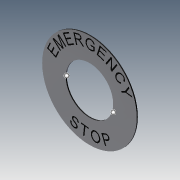
# Autodesk Inventor part: E-Stop Collar
Saved by Autodesk Inventor 2016 (Build 200138000, 138)
## iProperties
Created: 2005-06-20
Part Number: E-Stop Collar
Checked By: ~
Material: Generic
Document SubType Name: Modeling
Designer: BassBW
Manufacturer: Standard
Standards Organization: Custom
Density: 1 g/cm^3
Appearance: Black
SCALE: 1:1
STOCK SIZE: SEE DWG
UNITS: ANSI
COMMODITY: MFG
Author: BassBW
Autodesk Inventor part; units mm, degrees
ref_plane "YZ Plane" through (0, 0, 0) normal (1, 0, 0) x (0, 1, 0)
ref_plane "XZ Plane" through (0, 0, 0) normal (0, 1, 0) x (-1, 0, 0)
ref_plane "XY Plane" through (0, 0, 0) normal (0, 0, 1) x (1, 0, 0)
sketch "Sketch1" plane through (0, 0, 0) normal (0, 0, 1) x (1, 0, 0)
  circle A0 centre (0, 0) radius 29.972
  circle A1 centre (0, 0) radius 15
  dimension "d34" = 30
  dimension "d35" = 59.944
  constraints: 2 centre point, 2 coincident
  measures "d34" diameter of A1
  measures "d35" diameter of A0
extrude "Extrusion6" add sketch "Sketch1" along normal blind 0.635
sketch "Sketch10" plane through (0, 0, 0.635) normal (0, 0, 1) x (1, 0, 0)
  circle A0 centre (0, 0) radius 15 projected
  circle A1 centre (0, 0) radius 29.972 projected
  line L0 (0, 0) -> (0, 29.972) construction
  line L1 (0, 0) -> (-7.7573, 28.9507) construction
  line L2 (0, 0) -> (-14.986, 25.9565) construction
  line L3 (0, 0) -> (-21.1934, 21.1934) construction
  line L4 (0, 0) -> (-25.9565, 14.986) construction
  line L5 (0, 0) -> (-28.9507, 7.7573) construction
  line L6 (0, 0) -> (-29.972, 0) construction
  line L7 (0, 0) -> (-28.9507, -7.7573) construction
  line L8 (0, 0) -> (-25.9565, -14.986) construction
  line L9 (0, 0) -> (-21.1934, -21.1934) construction
  line L10 (0, 0) -> (-14.986, -25.9565) construction
  line L11 (0, 0) -> (-7.7573, -28.9507) construction
  line L12 (0, 0) -> (0, -29.972) construction
  line L13 (0, 0) -> (7.7573, -28.9507) construction
  line L14 (0, 0) -> (14.986, -25.9565) construction
  line L15 (0, 0) -> (21.1934, -21.1934) construction
  line L16 (0, 0) -> (25.9565, -14.986) construction
  line L17 (0, 0) -> (28.9507, -7.7573) construction
  line L18 (0, 0) -> (29.972, 0) construction
  line L19 (0, 0) -> (28.9507, 7.7573) construction
  line L20 (0, 0) -> (25.9565, 14.986) construction
  line L21 (0, 0) -> (21.1934, 21.1934) construction
  line L22 (0, 0) -> (14.986, 25.9565) construction
  line L23 (0, 0) -> (7.7573, 28.9507) construction
  circle A2 centre (0, 0) radius 20.6375 construction
  circle A3 centre (97.2399, -75.8106) radius 22.225 construction
  line L24 (-21.1834, 7.1074) -> (-26.9712, 9.7195)
  line L25 (-26.9712, 9.7195) -> (-25.1162, 13.8297)
  line L26 (-25.1162, 13.8297) -> (-24.4452, 13.5269)
  line L27 (-24.4452, 13.5269) -> (-25.9595, 10.1716)
  line L28 (-25.9595, 10.1716) -> (-24.1979, 9.3766)
  line L29 (-24.1979, 9.3766) -> (-22.7972, 12.4802)
  line L30 (-22.7972, 12.4802) -> (-22.1262, 12.1774)
  line L31 (-22.1262, 12.1774) -> (-23.5269, 9.0737)
  line L32 (-23.5269, 9.0737) -> (-21.5137, 8.1652)
  line L33 (-21.5137, 8.1652) -> (-19.9237, 11.6882)
  line L34 (-19.9237, 11.6882) -> (-19.2527, 11.3853)
  line L35 (-19.2527, 11.3853) -> (-21.1834, 7.1074)
  line L36 (-18.6254, 12.3234) -> (-23.3979, 16.5122)
  line L37 (-23.3979, 16.5122) -> (-22.5442, 17.4849)
  line L38 (-22.5442, 17.4849) -> (-18.2473, 15.5924)
  spline S0 degree 4 poles (-18.2473, 15.5924) (-18.2111, 15.5763) (-18.1401, 15.5449) (-18.0377, 15.4993) (-17.9095, 15.4421) (-17.7897, 15.3882) (-17.6783, 15.3378) (-17.5753, 15.2907) (-17.4806, 15.2471) (-17.4158, 15.217) (-17.3755, 15.198) (-17.356, 15.1888) knots 0 0 0 0 0 0.125 0.25 0.375 0.5 0.625 0.75 0.875 1 1 1 1 1
  spline S1 degree 4 poles (-17.356, 15.1888) (-17.3753, 15.1977) (-17.4137, 15.2188) (-17.4704, 15.2599) (-17.544, 15.3341) (-17.6157, 15.4274) (-17.6854, 15.5401) (-17.7533, 15.672) (-17.8191, 15.8231) (-17.8671, 15.9509) (-17.8984, 16.0425) (-17.9139, 16.0899) knots 0 0 0 0 0 0.125 0.25 0.375 0.5 0.625 0.75 0.875 1 1 1 1 1
  line L39 (-17.9139, 16.0899) -> (-20.3046, 20.0365)
  line L40 (-20.3046, 20.0365) -> (-19.4519, 21.008)
  line L41 (-19.4519, 21.008) -> (-14.6794, 16.8192)
  line L42 (-14.6794, 16.8192) -> (-15.2258, 16.1967)
  line L43 (-15.2258, 16.1967) -> (-19.3066, 19.7785)
  line L44 (-19.3066, 19.7785) -> (-16.3432, 14.9236)
  line L45 (-16.3432, 14.9236) -> (-16.9626, 14.2179)
  line L46 (-16.9626, 14.2179) -> (-22.1598, 16.5277)
  line L47 (-22.1598, 16.5277) -> (-18.079, 12.9459)
  line L48 (-18.079, 12.9459) -> (-18.6254, 12.3234)
  line L49 (-13.6101, 17.7205) -> (-16.9547, 23.1183)
  line L50 (-16.9547, 23.1183) -> (-13.1215, 25.4934)
  line L51 (-13.1215, 25.4934) -> (-12.7337, 24.8676)
  line L52 (-12.7337, 24.8676) -> (-15.8628, 22.9287)
  line L53 (-15.8628, 22.9287) -> (-14.8449, 21.2859)
  line L54 (-14.8449, 21.2859) -> (-11.9505, 23.0793)
  line L55 (-11.9505, 23.0793) -> (-11.5627, 22.4535)
  line L56 (-11.5627, 22.4535) -> (-14.4572, 20.66)
  line L57 (-14.4572, 20.66) -> (-13.2938, 18.7825)
  line L58 (-13.2938, 18.7825) -> (-10.0082, 20.8184)
  line L59 (-10.0082, 20.8184) -> (-9.6204, 20.1925)
  line L60 (-9.6204, 20.1925) -> (-13.6101, 17.7205)
  line L61 (-8.4915, 20.6592) -> (-10.2418, 26.7632)
  line L62 (-10.2418, 26.7632) -> (-7.6307, 27.5119)
  spline S2 degree 4 poles (-7.6307, 27.5119) (-7.5837, 27.5279) (-7.4887, 27.5575) (-7.3437, 27.5947) (-7.1453, 27.6296) (-6.9424, 27.6495) (-6.7362, 27.6533) (-6.529, 27.639) (-6.3241, 27.604) (-6.1251, 27.5462) (-5.936, 27.4647) (-5.7602, 27.361) (-5.6004, 27.2395) (-5.4589, 27.1057) (-5.3372, 26.9653) (-5.2365, 26.8227) (-5.1572, 26.6804) (-5.114, 26.5746) (-5.0925, 26.5046) (-5.0835, 26.4697) knots 0 0 0 0 0 0.0625 0.125 0.1875 0.25 0.3125 0.375 0.4375 0.5 0.5625 0.625 0.6875 0.75 0.8125 0.875 0.9375 1 1 1 1 1
  spline S3 degree 4 poles (-5.0835, 26.4697) (-5.0692, 26.4244) (-5.0454, 26.3325) (-5.0248, 26.1909) (-5.0273, 25.9947) (-5.0593, 25.7922) (-5.1197, 25.5855) (-5.2066, 25.3784) (-5.3175, 25.1763) (-5.4496, 24.9849) (-5.6002, 24.8093) (-5.7677, 24.6532) (-5.951, 24.5185) (-6.1001, 24.4343) (-6.2046, 24.3857) (-6.2581, 24.3632) knots 0 0 0 0 0 0.083333 0.166667 0.25 0.333333 0.416667 0.5 0.583333 0.666667 0.75 0.833333 0.916667 1 1 1 1 1
  spline S4 degree 4 poles (-6.2581, 24.3632) (-6.2373, 24.3584) (-6.1963, 24.3485) (-6.1368, 24.333) (-6.0616, 24.3112) (-5.9906, 24.2882) (-5.9236, 24.264) (-5.8608, 24.2386) (-5.802, 24.2121) (-5.7611, 24.1913) (-5.7351, 24.177) (-5.7225, 24.1698) knots 0 0 0 0 0 0.125 0.25 0.375 0.5 0.625 0.75 0.875 1 1 1 1 1
  spline S5 degree 4 poles (-5.7225, 24.1698) (-5.696, 24.1538) (-5.6431, 24.1213) (-5.5636, 24.0704) (-5.4573, 23.9985) (-5.3509, 23.9226) (-5.2442, 23.8427) (-5.1373, 23.7588) (-5.0302, 23.6708) (-4.9496, 23.6018) (-4.8959, 23.5544) (-4.869, 23.5304) knots 0 0 0 0 0 0.125 0.25 0.375 0.5 0.625 0.75 0.875 1 1 1 1 1
  line L63 (-4.869, 23.5304) -> (-3.3841, 22.1238)
  line L64 (-3.3841, 22.1238) -> (-4.2964, 21.8622)
  line L65 (-4.2964, 21.8622) -> (-5.4387, 22.9348)
  spline S6 degree 4 poles (-5.4387, 22.9348) (-5.4676, 22.9622) (-5.526, 23.017) (-5.6152, 23.0989) (-5.7369, 23.2072) (-5.8614, 23.3143) (-5.9881, 23.4194) (-6.1159, 23.5208) (-6.2435, 23.6163) (-6.369, 23.7031) (-6.4906, 23.7791) (-6.6065, 23.8426) (-6.7153, 23.8935) (-6.8159, 23.9324) (-6.9074, 23.9604) (-6.9893, 23.9785) (-7.0613, 23.9875) (-7.1077, 23.9875) (-7.1353, 23.9846) (-7.1482, 23.9823) knots 0 0 0 0 0 0.0625 0.125 0.1875 0.25 0.3125 0.375 0.4375 0.5 0.5625 0.625 0.6875 0.75 0.8125 0.875 0.9375 1 1 1 1 1
  spline S7 degree 4 poles (-7.1482, 23.9823) (-7.1586, 23.9798) (-7.1799, 23.9747) (-7.2135, 23.9667) (-7.2616, 23.9557) (-7.313, 23.9442) (-7.3677, 23.9322) (-7.4258, 23.9198) (-7.4871, 23.907) (-7.5356, 23.897) (-7.569, 23.8902) (-7.586, 23.8867) knots 0 0 0 0 0 0.125 0.25 0.375 0.5 0.625 0.75 0.875 1 1 1 1 1
  line L66 (-7.586, 23.8867) -> (-8.4817, 23.6299)
  line L67 (-8.4817, 23.6299) -> (-7.6953, 20.8875)
  line L68 (-7.6953, 20.8875) -> (-8.4915, 20.6592)
  line L69 (-8.6846, 24.3376) -> (-7.0245, 24.8136)
  spline S8 degree 4 poles (-7.0245, 24.8136) (-6.9917, 24.8213) (-6.9261, 24.8385) (-6.8282, 24.8693) (-6.6986, 24.9205) (-6.5704, 24.9818) (-6.445, 25.0533) (-6.3244, 25.1348) (-6.2119, 25.2263) (-6.1109, 25.3273) (-6.0242, 25.4364) (-5.9537, 25.5514) (-5.8999, 25.669) (-5.8623, 25.7854) (-5.8397, 25.8968) (-5.8313, 26.0006) (-5.8366, 26.0952) (-5.8507, 26.1588) (-5.8645, 26.1978) (-5.8726, 26.2165) knots 0 0 0 0 0 0.0625 0.125 0.1875 0.25 0.3125 0.375 0.4375 0.5 0.5625 0.625 0.6875 0.75 0.8125 0.875 0.9375 1 1 1 1 1
  spline S9 degree 4 poles (-5.8726, 26.2165) (-5.8806, 26.2463) (-5.9003, 26.3044) (-5.9407, 26.3873) (-6.0164, 26.4895) (-6.113, 26.5828) (-6.2292, 26.6666) (-6.3621, 26.7393) (-6.5079, 26.7989) (-6.6626, 26.8433) (-6.8226, 26.8706) (-6.9851, 26.8795) (-7.149, 26.8693) (-7.2724, 26.847) (-7.3548, 26.8256) (-7.396, 26.8133) knots 0 0 0 0 0 0.083333 0.166667 0.25 0.333333 0.416667 0.5 0.583333 0.666667 0.75 0.833333 0.916667 1 1 1 1 1
  line L70 (-7.396, 26.8133) -> (-9.2427, 26.2838)
  line L71 (-9.2427, 26.2838) -> (-8.6846, 24.3376)
  line L72 (0.6669, 24.634) -> (0.6809, 25.3701)
  line L73 (0.6809, 25.3701) -> (3.3493, 25.3194)
  line L74 (3.3493, 25.3194) -> (3.305, 22.9889)
  spline S10 degree 4 poles (3.305, 22.9889) (3.2625, 22.9569) (3.1749, 22.8937) (3.0352, 22.8014) (2.8324, 22.6835) (2.6141, 22.571) (2.3821, 22.4647) (2.1402, 22.3663) (1.8933, 22.2778) (1.6469, 22.2015) (1.4061, 22.1397) (1.1745, 22.0938) (0.9543, 22.0647) (0.7983, 22.0559) (0.6985, 22.0557) (0.6496, 22.0571) knots 0 0 0 0 0 0.083333 0.166667 0.25 0.333333 0.416667 0.5 0.583333 0.666667 0.75 0.833333 0.916667 1 1 1 1 1
  spline S11 degree 4 poles (0.6496, 22.0571) (0.5839, 22.0551) (0.4507, 22.0568) (0.2456, 22.0764) (-0.0381, 22.1364) (-0.3308, 22.2304) (-0.6292, 22.3583) (-0.9272, 22.5201) (-1.2169, 22.7155) (-1.4897, 22.9429) (-1.7378, 23.1991) (-1.9557, 23.4786) (-2.1405, 23.7734) (-2.291, 24.0752) (-2.4074, 24.3759) (-2.4897, 24.6698) (-2.5383, 24.9536) (-2.5495, 25.1579) (-2.5457, 25.2901) (-2.5409, 25.3552) knots 0 0 0 0 0 0.0625 0.125 0.1875 0.25 0.3125 0.375 0.4375 0.5 0.5625 0.625 0.6875 0.75 0.8125 0.875 0.9375 1 1 1 1 1
  spline S12 degree 4 poles (-2.5409, 25.3552) (-2.5425, 25.4202) (-2.5402, 25.5524) (-2.5206, 25.7569) (-2.4621, 26.042) (-2.3712, 26.3378) (-2.2477, 26.6409) (-2.0915, 26.945) (-1.9025, 27.2414) (-1.6819, 27.521) (-1.4324, 27.7755) (-1.1592, 27.9988) (-0.8697, 28.188) (-0.5722, 28.3417) (-0.2742, 28.4601) (0.0186, 28.5433) (0.303, 28.5915) (0.509, 28.6015) (0.643, 28.5966) (0.7091, 28.5912) knots 0 0 0 0 0 0.0625 0.125 0.1875 0.25 0.3125 0.375 0.4375 0.5 0.5625 0.625 0.6875 0.75 0.8125 0.875 0.9375 1 1 1 1 1
  spline S13 degree 4 poles (0.7091, 28.5912) (0.7554, 28.5917) (0.8495, 28.5899) (0.9953, 28.5783) (1.1987, 28.5451) (1.4103, 28.4942) (1.6279, 28.4251) (1.8477, 28.3376) (2.0645, 28.2311) (2.2726, 28.1058) (2.4667, 27.9625) (2.643, 27.8038) (2.7992, 27.6333) (2.9346, 27.4554) (3.0488, 27.2741) (3.1419, 27.0926) (3.214, 26.9124) (3.2522, 26.7789) (3.2707, 26.6907) (3.2782, 26.6468) knots 0 0 0 0 0 0.0625 0.125 0.1875 0.25 0.3125 0.375 0.4375 0.5 0.5625 0.625 0.6875 0.75 0.8125 0.875 0.9375 1 1 1 1 1
  line L75 (3.2782, 26.6468) -> (2.5123, 26.4542)
  spline S14 degree 4 poles (2.5123, 26.4542) (2.5056, 26.4862) (2.4899, 26.5504) (2.4597, 26.6473) (2.4058, 26.7773) (2.3383, 26.9079) (2.257, 27.0378) (2.1614, 27.165) (2.0514, 27.2868) (1.927, 27.4004) (1.7896, 27.5031) (1.6418, 27.5933) (1.4874, 27.6702) (1.3307, 27.7337) (1.1757, 27.7839) (1.0255, 27.8212) (0.8817, 27.8455) (0.7791, 27.8542) (0.7131, 27.8557) (0.6807, 27.8554) knots 0 0 0 0 0 0.0625 0.125 0.1875 0.25 0.3125 0.375 0.4375 0.5 0.5625 0.625 0.6875 0.75 0.8125 0.875 0.9375 1 1 1 1 1
  spline S15 degree 4 poles (0.6807, 27.8554) (0.6432, 27.8573) (0.5672, 27.859) (0.45, 27.8549) (0.2875, 27.8363) (0.1195, 27.8045) (-0.0528, 27.7596) (-0.2269, 27.7014) (-0.3994, 27.6299) (-0.5666, 27.5458) (-0.7247, 27.4499) (-0.8707, 27.3446) (-1.0028, 27.2328) (-1.1196, 27.1182) (-1.2206, 27.004) (-1.3054, 26.893) (-1.3738, 26.7864) (-1.4128, 26.7103) (-1.4333, 26.6614) (-1.4422, 26.6373) knots 0 0 0 0 0 0.0625 0.125 0.1875 0.25 0.3125 0.375 0.4375 0.5 0.5625 0.625 0.6875 0.75 0.8125 0.875 0.9375 1 1 1 1 1
  spline S16 degree 4 poles (-1.4422, 26.6373) (-1.4583, 26.6008) (-1.4893, 26.5272) (-1.5319, 26.4153) (-1.581, 26.2631) (-1.6224, 26.1079) (-1.6561, 25.9496) (-1.6822, 25.7883) (-1.7006, 25.6239) (-1.7087, 25.4984) (-1.7115, 25.4137) (-1.7122, 25.3711) knots 0 0 0 0 0 0.125 0.25 0.375 0.5 0.625 0.75 0.875 1 1 1 1 1
  spline S17 degree 4 poles (-1.7122, 25.3711) (-1.7163, 25.3156) (-1.7204, 25.2038) (-1.7142, 25.0334) (-1.6811, 24.8007) (-1.6231, 24.5636) (-1.5401, 24.3244) (-1.4316, 24.0873) (-1.2972, 23.8581) (-1.1377, 23.6431) (-0.9548, 23.4479) (-0.7528, 23.2766) (-0.5382, 23.1311) (-0.318, 23.0118) (-0.0992, 22.9183) (0.1131, 22.8502) (0.3158, 22.8071) (0.4598, 22.7935) (0.5522, 22.7927) (0.5974, 22.7944) knots 0 0 0 0 0 0.0625 0.125 0.1875 0.25 0.3125 0.375 0.4375 0.5 0.5625 0.625 0.6875 0.75 0.8125 0.875 0.9375 1 1 1 1 1
  spline S18 degree 4 poles (0.5974, 22.7944) (0.6354, 22.7941) (0.7128, 22.7956) (0.8335, 22.8043) (1.0033, 22.8289) (1.1812, 22.866) (1.3651, 22.9145) (1.5514, 22.9727) (1.7349, 23.038) (1.9102, 23.1074) (2.0719, 23.1784) (2.2161, 23.249) (2.3407, 23.318) (2.4188, 23.3682) (2.4639, 23.401) (2.4847, 23.4172) knots 0 0 0 0 0 0.083333 0.166667 0.25 0.333333 0.416667 0.5 0.583333 0.666667 0.75 0.833333 0.916667 1 1 1 1 1
  line L76 (2.4847, 23.4172) -> (2.5072, 24.599)
  line L77 (2.5072, 24.599) -> (0.6669, 24.634)
  line L78 (4.5777, 21.87) -> (6.494, 27.9239)
  line L79 (6.494, 27.9239) -> (10.7932, 26.563)
  line L80 (10.7932, 26.563) -> (10.571, 25.8611)
  line L81 (10.571, 25.8611) -> (7.0614, 26.972)
  line L82 (7.0614, 26.972) -> (6.4782, 25.1295)
  line L83 (6.4782, 25.1295) -> (9.7245, 24.1019)
  line L84 (9.7245, 24.1019) -> (9.5023, 23.4)
  line L85 (9.5023, 23.4) -> (6.256, 24.4276)
  line L86 (6.256, 24.4276) -> (5.5895, 22.3219)
  line L87 (5.5895, 22.3219) -> (9.2745, 21.1554)
  line L88 (9.2745, 21.1554) -> (9.0523, 20.4535)
  line L89 (9.0523, 20.4535) -> (4.5777, 21.87)
  line L90 (10.1418, 19.901) -> (13.6325, 25.2055)
  line L91 (13.6325, 25.2055) -> (14.3689, 24.721)
  line L92 (14.3689, 24.721) -> (14.3133, 18.8739)
  line L93 (14.3133, 18.8739) -> (17.0151, 22.9796)
  line L94 (17.0151, 22.9796) -> (17.707, 22.5243)
  line L95 (17.707, 22.5243) -> (14.2163, 17.2198)
  line L96 (14.2163, 17.2198) -> (13.4799, 17.7043)
  line L97 (13.4799, 17.7043) -> (13.5355, 23.5514)
  line L98 (13.5355, 23.5514) -> (10.8337, 19.4457)
  line L99 (10.8337, 19.4457) -> (10.1418, 19.901)
  line L100 (19.8442, 14.3837) -> (20.2195, 13.6161)
  spline S19 degree 4 poles (20.2195, 13.6161) (20.1553, 13.5829) (20.0244, 13.5217) (19.8209, 13.4461) (19.5351, 13.3772) (19.2365, 13.3403) (18.9278, 13.3346) (18.6145, 13.3595) (18.3041, 13.4135) (18.0049, 13.4952) (17.7245, 13.6034) (17.4684, 13.7371) (17.2398, 13.8958) (17.0899, 14.0334) (16.9996, 14.1333) (16.9569, 14.1854) knots 0 0 0 0 0 0.083333 0.166667 0.25 0.333333 0.416667 0.5 0.583333 0.666667 0.75 0.833333 0.916667 1 1 1 1 1
  spline S20 degree 4 poles (16.9569, 14.1854) (16.9098, 14.2339) (16.8201, 14.3354) (16.699, 14.5007) (16.5646, 14.747) (16.4579, 15.0182) (16.3804, 15.3122) (16.3346, 15.6249) (16.324, 15.9508) (16.3508, 16.2833) (16.4157, 16.6155) (16.516, 16.9404) (16.6459, 17.2517) (16.7984, 17.5441) (16.9662, 17.8129) (17.1442, 18.0553) (17.3294, 18.2693) (17.4728, 18.4082) (17.5702, 18.491) (17.6194, 18.53) knots 0 0 0 0 0 0.0625 0.125 0.1875 0.25 0.3125 0.375 0.4375 0.5 0.5625 0.625 0.6875 0.75 0.8125 0.875 0.9375 1 1 1 1 1
  spline S21 degree 4 poles (17.6194, 18.53) (17.668, 18.575) (17.7694, 18.6624) (17.9344, 18.7851) (18.18, 18.9321) (18.4503, 19.0616) (18.7432, 19.1716) (19.0551, 19.2586) (19.3807, 19.3178) (19.7136, 19.3448) (20.0468, 19.3368) (20.373, 19.2937) (20.6851, 19.2186) (20.9768, 19.1166) (21.2427, 18.993) (21.4789, 18.852) (21.6834, 18.696) (21.8123, 18.5685) (21.8872, 18.4789) (21.922, 18.433) knots 0 0 0 0 0 0.0625 0.125 0.1875 0.25 0.3125 0.375 0.4375 0.5 0.5625 0.625 0.6875 0.75 0.8125 0.875 0.9375 1 1 1 1 1
  spline S22 degree 4 poles (21.922, 18.433) (21.9634, 18.3857) (22.042, 18.2874) (22.1471, 18.1291) (22.2616, 17.8966) (22.3506, 17.6439) (22.414, 17.3738) (22.4517, 17.0914) (22.4634, 16.8038) (22.4491, 16.5186) (22.4086, 16.243) (22.3419, 15.9821) (22.2488, 15.7386) (22.1592, 15.57) (22.0907, 15.4639) (22.0542, 15.4124) knots 0 0 0 0 0 0.083333 0.166667 0.25 0.333333 0.416667 0.5 0.583333 0.666667 0.75 0.833333 0.916667 1 1 1 1 1
  line L101 (22.0542, 15.4124) -> (21.3717, 15.9197)
  spline S23 degree 4 poles (21.3717, 15.9197) (21.3985, 15.9587) (21.449, 16.0383) (21.5155, 16.1625) (21.5856, 16.3374) (21.6373, 16.5208) (21.6705, 16.7111) (21.6853, 16.9052) (21.6819, 17.099) (21.6603, 17.2878) (21.6205, 17.4674) (21.5628, 17.6344) (21.4871, 17.7873) (21.4169, 17.8908) (21.364, 17.9548) (21.3361, 17.9855) knots 0 0 0 0 0 0.083333 0.166667 0.25 0.333333 0.416667 0.5 0.583333 0.666667 0.75 0.833333 0.916667 1 1 1 1 1
  spline S24 degree 4 poles (21.3361, 17.9855) (21.3077, 18.0237) (21.2469, 18.0971) (21.1436, 18.1987) (20.9819, 18.3167) (20.797, 18.4167) (20.5906, 18.4976) (20.3662, 18.5568) (20.1282, 18.5917) (19.882, 18.5996) (19.6336, 18.5798) (19.3884, 18.5338) (19.1516, 18.4659) (18.9279, 18.3812) (18.7207, 18.285) (18.5327, 18.1815) (18.3653, 18.0727) (18.2555, 17.988) (18.1895, 17.9302) (18.1582, 17.9009) knots 0 0 0 0 0 0.0625 0.125 0.1875 0.25 0.3125 0.375 0.4375 0.5 0.5625 0.625 0.6875 0.75 0.8125 0.875 0.9375 1 1 1 1 1
  spline S25 degree 4 poles (18.1582, 17.9009) (18.117, 17.8691) (18.0354, 17.8021) (17.9161, 17.6918) (17.763, 17.5253) (17.6169, 17.3397) (17.4799, 17.1361) (17.3557, 16.9166) (17.2496, 16.6839) (17.1667, 16.4419) (17.1112, 16.1951) (17.0849, 15.9491) (17.0865, 15.7095) (17.1131, 15.4823) (17.161, 15.2725) (17.2272, 15.084) (17.31, 14.9188) (17.3841, 14.8131) (17.4387, 14.7508) (17.4674, 14.7217) knots 0 0 0 0 0 0.0625 0.125 0.1875 0.25 0.3125 0.375 0.4375 0.5 0.5625 0.625 0.6875 0.75 0.8125 0.875 0.9375 1 1 1 1 1
  spline S26 degree 4 poles (17.4674, 14.7217) (17.4974, 14.6848) (17.5611, 14.614) (17.6679, 14.517) (17.8321, 14.406) (18.0173, 14.3136) (18.2212, 14.2401) (18.4395, 14.1863) (18.6665, 14.1531) (18.896, 14.1417) (19.1223, 14.1529) (19.3415, 14.1876) (19.5512, 14.2461) (19.7008, 14.3079) (19.797, 14.3571) (19.8442, 14.3837) knots 0 0 0 0 0 0.083333 0.166667 0.25 0.333333 0.416667 0.5 0.583333 0.666667 0.75 0.833333 0.916667 1 1 1 1 1
  line L102 (20.0309, 9.6686) -> (22.4765, 10.7899)
  line L103 (22.4765, 10.7899) -> (24.8059, 14.4901)
  line L104 (24.8059, 14.4901) -> (25.2104, 13.6078)
  line L105 (25.2104, 13.6078) -> (23.99, 11.6705)
  spline S27 degree 4 poles (23.99, 11.6705) (23.9679, 11.6348) (23.9242, 11.5644) (23.86, 11.461) (23.777, 11.3281) (23.6966, 11.1999) (23.6189, 11.0765) (23.5439, 10.9578) (23.4716, 10.844) (23.4193, 10.7622) (23.3853, 10.7093) (23.3686, 10.6832) knots 0 0 0 0 0 0.125 0.25 0.375 0.5 0.625 0.75 0.875 1 1 1 1 1
  spline S28 degree 4 poles (23.3686, 10.6832) (23.3977, 10.6782) (23.4572, 10.6682) (23.5508, 10.6534) (23.684, 10.6341) (23.8256, 10.6153) (23.9756, 10.5968) (24.1341, 10.5789) (24.3009, 10.5613) (24.4324, 10.5485) (24.5228, 10.54) (24.5688, 10.5359) knots 0 0 0 0 0 0.125 0.25 0.375 0.5 0.625 0.75 0.875 1 1 1 1 1
  line L106 (24.5688, 10.5359) -> (26.741, 10.2695)
  line L107 (26.741, 10.2695) -> (27.1455, 9.3871)
  line L108 (27.1455, 9.3871) -> (22.8217, 10.037)
  line L109 (22.8217, 10.037) -> (20.3761, 8.9157)
  line L110 (20.3761, 8.9157) -> (20.0309, 9.6686)
  circle A4 centre (97.2399, -80.7117) radius 22.225 construction
  line L111 (-12.1327, -22.3139) -> (-11.351, -22.5876)
  spline S29 degree 4 poles (-11.351, -22.5876) (-11.3611, -22.6199) (-11.379, -22.6859) (-11.3987, -22.7891) (-11.4105, -22.935) (-11.4076, -23.0886) (-11.3893, -23.2488) (-11.3544, -23.4132) (-11.3012, -23.5788) (-11.2288, -23.742) (-11.1374, -23.8992) (-11.0289, -24.0474) (-10.9072, -24.1839) (-10.7766, -24.3069) (-10.6417, -24.4147) (-10.5054, -24.5064) (-10.3697, -24.5816) (-10.2688, -24.6253) (-10.2021, -24.6488) (-10.1688, -24.6591) knots 0 0 0 0 0 0.0625 0.125 0.1875 0.25 0.3125 0.375 0.4375 0.5 0.5625 0.625 0.6875 0.75 0.8125 0.875 0.9375 1 1 1 1 1
  spline S30 degree 4 poles (-10.1688, -24.6591) (-10.1411, -24.6702) (-10.0842, -24.6908) (-9.9943, -24.7169) (-9.8652, -24.7423) (-9.7277, -24.7579) (-9.5829, -24.7633) (-9.4333, -24.7575) (-9.2823, -24.7393) (-9.1336, -24.7075) (-8.9912, -24.662) (-8.8587, -24.6038) (-8.7387, -24.5355) (-8.6333, -24.4602) (-8.5439, -24.3813) (-8.4716, -24.3014) (-8.4168, -24.2218) (-8.3891, -24.1628) (-8.3766, -24.1239) (-8.3718, -24.1045) knots 0 0 0 0 0 0.0625 0.125 0.1875 0.25 0.3125 0.375 0.4375 0.5 0.5625 0.625 0.6875 0.75 0.8125 0.875 0.9375 1 1 1 1 1
  spline S31 degree 4 poles (-8.3718, -24.1045) (-8.3646, -24.0864) (-8.3521, -24.0491) (-8.3391, -23.9903) (-8.3333, -23.906) (-8.3389, -23.8163) (-8.3555, -23.722) (-8.3826, -23.6247) (-8.4194, -23.5268) (-8.4649, -23.4304) (-8.5185, -23.3379) (-8.5794, -23.2508) (-8.6475, -23.1699) (-8.7038, -23.1141) (-8.7436, -23.0791) (-8.7641, -23.0622) knots 0 0 0 0 0 0.083333 0.166667 0.25 0.333333 0.416667 0.5 0.583333 0.666667 0.75 0.833333 0.916667 1 1 1 1 1
  spline S32 degree 4 poles (-8.7641, -23.0622) (-8.7846, -23.0459) (-8.8302, -23.0107) (-8.9122, -22.9494) (-9.0483, -22.8509) (-9.2096, -22.7368) (-9.3924, -22.6089) (-9.5899, -22.4711) (-9.7932, -22.3284) (-9.9926, -22.1862) (-10.1792, -22.0493) (-10.3466, -21.9215) (-10.4911, -21.8048) (-10.5813, -21.7261) (-10.6332, -21.6776) (-10.6571, -21.6544) knots 0 0 0 0 0 0.083333 0.166667 0.25 0.333333 0.416667 0.5 0.583333 0.666667 0.75 0.833333 0.916667 1 1 1 1 1
  spline S33 degree 4 poles (-10.6571, -21.6544) (-10.681, -21.6298) (-10.7275, -21.5786) (-10.7925, -21.4962) (-10.8699, -21.375) (-10.9379, -21.2431) (-10.9961, -21.1018) (-11.044, -20.9538) (-11.0808, -20.8026) (-11.1056, -20.652) (-11.1177, -20.5057) (-11.1164, -20.3663) (-11.1014, -20.2352) (-11.0798, -20.1435) (-11.0607, -20.0855) (-11.0501, -20.0572) knots 0 0 0 0 0 0.083333 0.166667 0.25 0.333333 0.416667 0.5 0.583333 0.666667 0.75 0.833333 0.916667 1 1 1 1 1
  spline S34 degree 4 poles (-11.0501, -20.0572) (-11.041, -20.0238) (-11.0187, -19.9572) (-10.9725, -19.8576) (-10.8853, -19.7256) (-10.7731, -19.5953) (-10.6368, -19.4687) (-10.4779, -19.3494) (-10.299, -19.2419) (-10.1032, -19.1507) (-9.8947, -19.0793) (-9.6785, -19.029) (-9.4602, -18.9993) (-9.2451, -18.9883) (-9.0379, -18.994) (-8.8421, -19.0147) (-8.6593, -19.0496) (-8.5327, -19.086) (-8.453, -19.1149) (-8.4144, -19.1305) knots 0 0 0 0 0 0.0625 0.125 0.1875 0.25 0.3125 0.375 0.4375 0.5 0.5625 0.625 0.6875 0.75 0.8125 0.875 0.9375 1 1 1 1 1
  spline S35 degree 4 poles (-8.4144, -19.1305) (-8.3705, -19.1435) (-8.2827, -19.1731) (-8.1504, -19.2279) (-7.973, -19.3214) (-7.7956, -19.4354) (-7.6201, -19.5694) (-7.4504, -19.7227) (-7.2915, -19.8939) (-7.1488, -20.0812) (-7.027, -20.2814) (-6.929, -20.4905) (-6.8555, -20.703) (-6.806, -20.9132) (-6.7792, -21.1161) (-6.7739, -21.3078) (-6.7895, -21.4861) (-6.8166, -21.6092) (-6.8416, -21.6864) (-6.8557, -21.7238) knots 0 0 0 0 0 0.0625 0.125 0.1875 0.25 0.3125 0.375 0.4375 0.5 0.5625 0.625 0.6875 0.75 0.8125 0.875 0.9375 1 1 1 1 1
  line L112 (-6.8557, -21.7238) -> (-7.6375, -21.4501)
  spline S36 degree 4 poles (-7.6375, -21.4501) (-7.6264, -21.4105) (-7.6083, -21.3309) (-7.5935, -21.2106) (-7.5983, -21.0485) (-7.6273, -20.8854) (-7.6797, -20.7226) (-7.7537, -20.5628) (-7.8473, -20.4098) (-7.958, -20.2675) (-8.0838, -20.1395) (-8.2229, -20.0284) (-8.3747, -19.9355) (-8.4977, -19.8801) (-8.5838, -19.8495) (-8.6278, -19.8358) knots 0 0 0 0 0 0.083333 0.166667 0.25 0.333333 0.416667 0.5 0.583333 0.666667 0.75 0.833333 0.916667 1 1 1 1 1
  spline S37 degree 4 poles (-8.6278, -19.8358) (-8.6709, -19.8196) (-8.7573, -19.7904) (-8.8869, -19.7565) (-9.0597, -19.7307) (-9.2318, -19.7242) (-9.4018, -19.7363) (-9.5667, -19.7658) (-9.7227, -19.811) (-9.8653, -19.8702) (-9.9901, -19.9416) (-10.0941, -20.0238) (-10.1755, -20.1162) (-10.219, -20.1929) (-10.2402, -20.2473) (-10.2488, -20.2753) knots 0 0 0 0 0 0.083333 0.166667 0.25 0.333333 0.416667 0.5 0.583333 0.666667 0.75 0.833333 0.916667 1 1 1 1 1
  spline S38 degree 4 poles (-10.2488, -20.2753) (-10.2559, -20.2954) (-10.2687, -20.3355) (-10.2838, -20.395) (-10.2957, -20.4733) (-10.2995, -20.5504) (-10.295, -20.6264) (-10.2824, -20.7013) (-10.2616, -20.7751) (-10.2399, -20.8296) (-10.2227, -20.8655) (-10.2134, -20.8834) knots 0 0 0 0 0 0.125 0.25 0.375 0.5 0.625 0.75 0.875 1 1 1 1 1
  spline S39 degree 4 poles (-10.2134, -20.8834) (-10.1946, -20.9084) (-10.1511, -20.9609) (-10.0687, -21.047) (-9.9246, -21.1762) (-9.7483, -21.3189) (-9.5443, -21.473) (-9.3206, -21.6346) (-9.0883, -21.7985) (-8.8589, -21.9591) (-8.6432, -22.1114) (-8.449, -22.2515) (-8.2806, -22.3774) (-8.175, -22.4606) (-8.114, -22.5109) (-8.0858, -22.5348) knots 0 0 0 0 0 0.083333 0.166667 0.25 0.333333 0.416667 0.5 0.583333 0.666667 0.75 0.833333 0.916667 1 1 1 1 1
  spline S40 degree 4 poles (-8.0858, -22.5348) (-8.0561, -22.5623) (-7.9985, -22.6193) (-7.9177, -22.7114) (-7.8212, -22.8471) (-7.7359, -22.9951) (-7.6624, -23.1537) (-7.6013, -23.3203) (-7.5538, -23.491) (-7.5208, -23.6614) (-7.5036, -23.8278) (-7.5027, -23.987) (-7.5187, -24.1377) (-7.5435, -24.2437) (-7.5657, -24.3113) (-7.5782, -24.3443) knots 0 0 0 0 0 0.083333 0.166667 0.25 0.333333 0.416667 0.5 0.583333 0.666667 0.75 0.833333 0.916667 1 1 1 1 1
  spline S41 degree 4 poles (-7.5782, -24.3443) (-7.588, -24.3793) (-7.612, -24.4494) (-7.6616, -24.5544) (-7.7547, -24.694) (-7.8745, -24.8323) (-8.0198, -24.9673) (-8.1889, -25.0954) (-8.3791, -25.2118) (-8.5869, -25.3119) (-8.8081, -25.3919) (-9.0372, -25.4503) (-9.2686, -25.4873) (-9.4966, -25.5042) (-9.7163, -25.5027) (-9.9245, -25.4843) (-10.119, -25.4497) (-10.2542, -25.4119) (-10.3395, -25.3815) (-10.3809, -25.3649) knots 0 0 0 0 0 0.0625 0.125 0.1875 0.25 0.3125 0.375 0.4375 0.5 0.5625 0.625 0.6875 0.75 0.8125 0.875 0.9375 1 1 1 1 1
  spline S42 degree 4 poles (-10.3809, -25.3649) (-10.4341, -25.3493) (-10.5404, -25.3141) (-10.6988, -25.2496) (-10.9081, -25.1399) (-11.1146, -25.0069) (-11.3159, -24.8509) (-11.5083, -24.6726) (-11.6862, -24.4732) (-11.8442, -24.2547) (-11.9772, -24.0204) (-12.0826, -23.7752) (-12.1599, -23.5252) (-12.2101, -23.2773) (-12.2349, -23.0374) (-12.2357, -22.8101) (-12.2135, -22.598) (-12.1797, -22.4511) (-12.1496, -22.3587) (-12.1327, -22.3139) knots 0 0 0 0 0 0.0625 0.125 0.1875 0.25 0.3125 0.375 0.4375 0.5 0.5625 0.625 0.6875 0.75 0.8125 0.875 0.9375 1 1 1 1 1
  line L113 (-4.0735, -26.7652) -> (-3.4252, -21.189)
  line L114 (-3.4252, -21.189) -> (-5.5277, -20.9446)
  line L115 (-5.5277, -20.9446) -> (-5.4426, -20.2133)
  line L116 (-5.4426, -20.2133) -> (-0.4149, -20.7978)
  line L117 (-0.4149, -20.7978) -> (-0.4999, -21.5291)
  line L118 (-0.4999, -21.5291) -> (-2.6024, -21.2847)
  line L119 (-2.6024, -21.2847) -> (-3.2508, -26.8609)
  line L120 (-3.2508, -26.8609) -> (-4.0735, -26.7652)
  spline S43 degree 4 poles (0.872, -23.9984) (0.8563, -23.8936) (0.8342, -23.6845) (0.8293, -23.372) (0.8788, -22.9581) (0.9832, -22.5485) (1.14, -22.1473) (1.3442, -21.7614) (1.5893, -21.4007) (1.8677, -21.0762) (2.1726, -20.7979) (2.499, -20.5734) (2.844, -20.4067) (3.1158, -20.3264) (3.3028, -20.2929) (3.3977, -20.2811) knots 0 0 0 0 0 0.083333 0.166667 0.25 0.333333 0.416667 0.5 0.583333 0.666667 0.75 0.833333 0.916667 1 1 1 1 1
  spline S44 degree 4 poles (3.3977, -20.2811) (3.4582, -20.27) (3.5816, -20.2533) (3.7739, -20.2453) (4.0443, -20.2686) (4.3274, -20.3259) (4.62, -20.4173) (4.9166, -20.5431) (5.2096, -20.7031) (5.4909, -20.8961) (5.753, -21.1194) (5.9903, -21.3679) (6.1994, -21.6344) (6.3785, -21.911) (6.5267, -22.1907) (6.6436, -22.468) (6.7291, -22.74) (6.7696, -22.9391) (6.786, -23.0696) (6.7916, -23.1343) knots 0 0 0 0 0 0.0625 0.125 0.1875 0.25 0.3125 0.375 0.4375 0.5 0.5625 0.625 0.6875 0.75 0.8125 0.875 0.9375 1 1 1 1 1
  spline S45 degree 4 poles (6.7916, -23.1343) (6.8033, -23.199) (6.8216, -23.3309) (6.8343, -23.536) (6.8216, -23.8235) (6.7789, -24.1239) (6.7059, -24.4341) (6.6018, -24.7489) (6.4656, -25.0608) (6.2975, -25.3617) (6.0992, -25.6438) (5.8752, -25.9005) (5.6322, -26.1276) (5.3783, -26.3222) (5.121, -26.4828) (4.8661, -26.6082) (4.6169, -26.6981) (4.4352, -26.7387) (4.3166, -26.7537) (4.2579, -26.7583) knots 0 0 0 0 0 0.0625 0.125 0.1875 0.25 0.3125 0.375 0.4375 0.5 0.5625 0.625 0.6875 0.75 0.8125 0.875 0.9375 1 1 1 1 1
  spline S46 degree 4 poles (4.2579, -26.7583) (4.1968, -26.7695) (4.0723, -26.7862) (3.8789, -26.7942) (3.608, -26.7704) (3.3253, -26.7124) (3.0336, -26.6201) (2.7384, -26.4937) (2.4468, -26.3338) (2.1667, -26.1418) (1.9053, -25.9209) (1.6683, -25.6766) (1.4594, -25.4164) (1.2804, -25.1482) (1.1326, -24.8796) (1.0163, -24.6161) (0.9319, -24.361) (0.8926, -24.1768) (0.8771, -24.0573) (0.872, -23.9984) knots 0 0 0 0 0 0.0625 0.125 0.1875 0.25 0.3125 0.375 0.4375 0.5 0.5625 0.625 0.6875 0.75 0.8125 0.875 0.9375 1 1 1 1 1
  spline S47 degree 4 poles (1.6943, -23.8988) (1.7034, -23.9747) (1.728, -24.1245) (1.7845, -24.3433) (1.8991, -24.6231) (2.0515, -24.89) (2.2391, -25.1416) (2.4568, -25.3739) (2.6979, -25.5811) (2.9544, -25.7568) (3.2194, -25.8952) (3.4875, -25.9919) (3.7559, -26.0444) (3.9564, -26.05) (4.0897, -26.0386) (4.1562, -26.0291) knots 0 0 0 0 0 0.083333 0.166667 0.25 0.333333 0.416667 0.5 0.583333 0.666667 0.75 0.833333 0.916667 1 1 1 1 1
  spline S48 degree 4 poles (4.1562, -26.0291) (4.2244, -26.021) (4.3588, -25.9971) (4.5545, -25.9386) (4.8031, -25.8154) (5.0386, -25.6483) (5.2589, -25.4404) (5.4602, -25.1974) (5.6372, -24.9268) (5.7845, -24.6367) (5.897, -24.3346) (5.9711, -24.0257) (6.005, -23.7129) (5.9995, -23.4762) (5.982, -23.3176) (5.9699, -23.2381) knots 0 0 0 0 0 0.083333 0.166667 0.25 0.333333 0.416667 0.5 0.583333 0.666667 0.75 0.833333 0.916667 1 1 1 1 1
  spline S49 degree 4 poles (5.9699, -23.2381) (5.9655, -23.1875) (5.9531, -23.0855) (5.9233, -22.9299) (5.8611, -22.7176) (5.7766, -22.5014) (5.6697, -22.2835) (5.5406, -22.0679) (5.3894, -21.8603) (5.2172, -21.6667) (5.0263, -21.4926) (4.8207, -21.3422) (4.6061, -21.2175) (4.3886, -21.1194) (4.1743, -21.048) (3.9676, -21.0029) (3.771, -20.984) (3.6319, -20.9895) (3.5429, -21.0019) (3.4993, -21.0103) knots 0 0 0 0 0 0.0625 0.125 0.1875 0.25 0.3125 0.375 0.4375 0.5 0.5625 0.625 0.6875 0.75 0.8125 0.875 0.9375 1 1 1 1 1
  spline S50 degree 4 poles (3.4993, -21.0103) (3.433, -21.0168) (3.3018, -21.0376) (3.1097, -21.0919) (2.8631, -21.2104) (2.6272, -21.3738) (2.4045, -21.5794) (2.1997, -21.8222) (2.0188, -22.0956) (1.8684, -22.3926) (1.7544, -22.707) (1.6808, -23.0343) (1.6498, -23.3722) (1.6593, -23.6328) (1.6802, -23.8096) (1.6943, -23.8988) knots 0 0 0 0 0 0.083333 0.166667 0.25 0.333333 0.416667 0.5 0.583333 0.666667 0.75 0.833333 0.916667 1 1 1 1 1
  line L121 (9.8262, -25.5304) -> (7.4673, -19.6348)
  line L122 (7.4673, -19.6348) -> (9.6208, -18.7732)
  spline S51 degree 4 poles (9.6208, -18.7732) (9.6554, -18.7592) (9.7236, -18.7321) (9.8225, -18.6939) (9.9475, -18.6477) (10.0657, -18.6064) (10.1772, -18.5699) (10.2818, -18.5383) (10.3797, -18.5116) (10.448, -18.4951) (10.4913, -18.4858) (10.5123, -18.4815) knots 0 0 0 0 0 0.125 0.25 0.375 0.5 0.625 0.75 0.875 1 1 1 1 1
  spline S52 degree 4 poles (10.5123, -18.4815) (10.5418, -18.4732) (10.6023, -18.4588) (10.6975, -18.444) (10.8335, -18.438) (10.978, -18.4459) (11.1297, -18.4681) (11.2865, -18.5056) (11.4453, -18.5593) (11.6028, -18.6297) (11.7554, -18.7165) (11.9, -18.8176) (12.0339, -18.9297) (12.1551, -19.049) (12.262, -19.1718) (12.3534, -19.2952) (12.4289, -19.4179) (12.4733, -19.5088) (12.4974, -19.5689) (12.5081, -19.5988) knots 0 0 0 0 0 0.0625 0.125 0.1875 0.25 0.3125 0.375 0.4375 0.5 0.5625 0.625 0.6875 0.75 0.8125 0.875 0.9375 1 1 1 1 1
  spline S53 degree 4 poles (12.5081, -19.5988) (12.536, -19.6505) (12.5846, -19.7566) (12.6361, -19.9238) (12.662, -20.1624) (12.6457, -20.4151) (12.5884, -20.6784) (12.4923, -20.9459) (12.3603, -21.209) (12.1954, -21.4586) (12.0005, -21.6866) (11.7775, -21.8873) (11.5275, -22.0575) (11.3201, -22.1613) (11.173, -22.2199) (11.0972, -22.2465) knots 0 0 0 0 0 0.083333 0.166667 0.25 0.333333 0.416667 0.5 0.583333 0.666667 0.75 0.833333 0.916667 1 1 1 1 1
  line L123 (11.0972, -22.2465) -> (9.638, -22.8303)
  line L124 (9.638, -22.8303) -> (10.5952, -25.2227)
  line L125 (10.5952, -25.2227) -> (9.8262, -25.5304)
  line L126 (9.3645, -22.1468) -> (10.8384, -21.557)
  spline S54 degree 4 poles (10.8384, -21.557) (10.8861, -21.5401) (10.9787, -21.5032) (11.1097, -21.4391) (11.2681, -21.336) (11.41, -21.216) (11.5348, -21.0806) (11.6409, -20.9328) (11.7266, -20.7765) (11.7898, -20.6161) (11.8283, -20.4559) (11.8409, -20.2989) (11.8267, -20.1468) (11.7957, -20.037) (11.7659, -19.9657) (11.7488, -19.9305) knots 0 0 0 0 0 0.083333 0.166667 0.25 0.333333 0.416667 0.5 0.583333 0.666667 0.75 0.833333 0.916667 1 1 1 1 1
  spline S55 degree 4 poles (11.7488, -19.9305) (11.7391, -19.905) (11.7175, -19.8545) (11.6788, -19.7806) (11.6144, -19.6859) (11.5379, -19.5952) (11.4504, -19.5095) (11.3538, -19.43) (11.2512, -19.3589) (11.1456, -19.2982) (11.0399, -19.25) (10.9365, -19.2158) (10.8363, -19.1964) (10.764, -19.1931) (10.7171, -19.196) (10.694, -19.1987) knots 0 0 0 0 0 0.083333 0.166667 0.25 0.333333 0.416667 0.5 0.583333 0.666667 0.75 0.833333 0.916667 1 1 1 1 1
  spline S56 degree 4 poles (10.694, -19.1987) (10.6798, -19.2) (10.6501, -19.2037) (10.6013, -19.212) (10.5276, -19.2289) (10.4454, -19.2516) (10.3546, -19.2802) (10.2552, -19.3146) (10.1473, -19.3549) (10.06, -19.3894) (9.9989, -19.4144) (9.9677, -19.4274) knots 0 0 0 0 0 0.125 0.25 0.375 0.5 0.625 0.75 0.875 1 1 1 1 1
  line L127 (9.9677, -19.4274) -> (8.5098, -20.0107)
  line L128 (8.5098, -20.0107) -> (9.3645, -22.1468)
  point P0 (-17.7248, 15.3588)
  point P1 (-17.6402, 15.4691)
  point P2 (-6.8234, 27.6502)
  point P3 (-5.9971, 27.4882)
  point P4 (-5.3736, 27.0044)
  point P5 (-5.0847, 25.7137)
  point P6 (-5.5165, 24.9101)
  point P7 (-5.955, 24.2751)
  point P8 (-5.3002, 23.8844)
  point P9 (-5.9655, 23.4)
  point P10 (-6.4969, 23.7809)
  point P11 (-6.9017, 23.9573)
  point P12 (-7.3387, 23.9386)
  point P13 (-6.4931, 25.027)
  point P14 (-6.0462, 25.4117)
  point P15 (-5.8467, 25.8699)
  point P16 (-6.1565, 26.612)
  point P17 (-6.7263, 26.8525)
  point P18 (2.502, 22.5207)
  point P19 (1.5043, 22.1661)
  point P20 (-0.4328, 22.2772)
  point P21 (-1.6143, 23.076)
  point P22 (-2.3659, 24.2769)
  point P23 (-2.3257, 26.4423)
  point P24 (-1.5491, 27.6518)
  point P25 (-0.3728, 28.4176)
  point P26 (1.5029, 28.4633)
  point P27 (2.3835, 28.0215)
  point P28 (3.0082, 27.3353)
  point P29 (2.3055, 26.9582)
  point P30 (1.8641, 27.4458)
  point P31 (1.2422, 27.7614)
  point P32 (0.0292, 27.7799)
  point P33 (-0.678, 27.4765)
  point P34 (-1.1961, 27.0299)
  point P35 (-1.6382, 26.0305)
  point P36 (-1.582, 24.451)
  point P37 (-1.0211, 23.5228)
  point P38 (-0.1594, 22.9465)
  point P39 (1.2781, 22.8923)
  point P40 (2.0168, 23.1549)
  point P41 (19.0813, 13.34)
  point P42 (17.8433, 13.5605)
  point P43 (16.4332, 15.1246)
  point P44 (16.3838, 16.4361)
  point P45 (16.9059, 17.7122)
  point P46 (18.5808, 19.1082)
  point P47 (19.9239, 19.3365)
  point P48 (21.1725, 19.022)
  point P49 (22.3772, 17.52)
  point P50 (22.4251, 16.3715)
  point P51 (21.6534, 16.6226)
  point P52 (21.6357, 17.3908)
  point P53 (20.7203, 18.4442)
  point P54 (19.7621, 18.5878)
  point P55 (18.7959, 18.3184)
  point P56 (17.547, 17.2331)
  point P57 (17.13, 16.265)
  point P58 (17.1529, 15.3206)
  point P59 (18.1018, 14.2853)
  point P60 (19.003, 14.1489)
  point P61 (23.6539, 11.1321)
  point P62 (23.8895, 10.6075)
  point P63 (-11.3995, -23.1479)
  point P64 (-11.1877, -23.8094)
  point P65 (-10.7001, -24.3665)
  point P66 (-9.6503, -24.7599)
  point P67 (-9.0323, -24.6734)
  point P68 (-8.5665, -24.3993)
  point P69 (-8.3466, -23.7778)
  point P70 (-8.4892, -23.39)
  point P71 (-9.2678, -22.6962)
  point P72 (-10.0984, -22.1082)
  point P73 (-10.9665, -21.1709)
  point P74 (-11.1114, -20.5686)
  point P75 (-10.7366, -19.5644)
  point P76 (-10.0308, -19.1282)
  point P77 (-9.1343, -18.9927)
  point P78 (-7.717, -19.4973)
  point P79 (-7.0757, -20.2056)
  point P80 (-6.7892, -21.0563)
  point P81 (-7.6522, -20.8143)
  point P82 (-8.0175, -20.2095)
  point P83 (-9.3418, -19.7337)
  point P84 (-9.9493, -19.9206)
  point P85 (-10.2965, -20.5888)
  point P86 (-9.6846, -21.366)
  point P87 (-8.7322, -22.0487)
  point P88 (-7.6989, -23.0778)
  point P89 (-7.5122, -23.7576)
  point P90 (-7.9115, -24.8635)
  point P91 (-8.6628, -25.337)
  point P92 (-9.6148, -25.5019)
  point P93 (-11.2064, -24.9334)
  point P94 (-11.9226, -24.1114)
  point P95 (-12.2251, -23.1096)
  point P96 (1.0716, -22.3339)
  point P97 (2.0586, -20.9085)
  point P98 (4.4138, -20.3562)
  point P99 (5.6035, -20.996)
  point P100 (6.4676, -22.0844)
  point P101 (6.7468, -24.2497)
  point P102 (6.1753, -25.53)
  point P103 (5.1871, -26.4377)
  point P104 (3.2281, -26.6785)
  point P105 (2.0358, -26.0274)
  point P106 (1.1813, -24.9627)
  point P107 (2.1549, -25.0236)
  point P108 (3.1185, -25.8387)
  point P109 (5.1178, -25.5685)
  point P110 (5.8305, -24.5039)
  point P111 (5.7269, -22.4038)
  point P112 (5.0971, -21.5605)
  point P113 (4.2346, -21.0707)
  point P114 (2.5609, -21.4406)
  point P115 (1.8318, -22.5048)
  point P116 (10.1297, -18.5857)
  point P117 (11.0322, -18.4551)
  point P118 (11.6697, -18.6693)
  point P119 (12.2162, -19.1209)
  point P120 (12.6243, -20.4953)
  point P121 (12.1231, -21.5378)
  point P122 (11.4842, -21.1326)
  point P123 (11.8114, -20.5167)
  point P124 (11.4923, -19.5519)
  point P125 (11.0848, -19.2716)
  point P126 (10.4084, -19.2636)
  point P127 (-17.3628, 15.1921)
  dimension "d40" = 360
  dimension "d42" = 41.275
  dimension "d43" = 44.45
  constraints: 258 end point, 3 centre point, 2 vertical alignment, 1 coincident, 1 equal radius, 1 vertical, 317 other
  measures "d42" diameter of A2
  measures "d43" diameter of A3
extrude "Extrusion7" add sketch "Sketch10" along normal blind 0.0254
body "Solid1"
